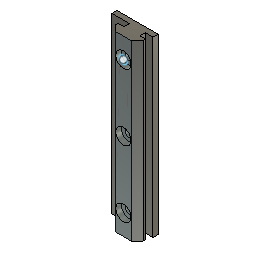
Slider v1 (Autodesk Fusion 360 design; units mm, degrees)
Autodesk Fusion 360 part; units mm, degrees
sketch "Sketch1" plane through (0, 0, 0) normal (0, 0, 1) x (1, 0, 0)
  line L0 (0, 0) -> (6.9, 0)
  line L1 (6.9, 0) -> (6.9, -2.1)
  line L2 (6.9, -2.1) -> (4.6, -2.1)
  line L3 (4.6, -2.1) -> (4.6, -3.1)
  line L4 (4.6, -3.1) -> (6.9335, -5.4335)
  line L5 (4.6, -3.1) -> (7.9, -3.1) construction
  line L6 (4.6, -2.1) -> (10.8, -2.1)
  line L7 (6.9, -2.1) -> (13.1, -2.1)
  line L8 (13.1, -2.1) -> (15.4, -2.1)
  line L9 (15.4, -2.1) -> (15.4, -3.1)
  line L10 (15.4, -3.1) -> (13.0665, -5.4335)
  line L11 (13.0665, -5.4335) -> (6.9335, -5.4335)
  line L12 (15.4, -2.1) -> (13.1, -2.1)
  line L13 (13.1, -2.1) -> (13.1, 0)
  line L14 (13.1, 0) -> (16.1, 0)
  line L15 (16.1, 0) -> (16.1, 2)
  line L16 (16.1, 2) -> (0, 2)
  line L17 (0, 2) -> (0, 0)
  dimension "d1" = 6.9
  dimension "d2" = 2.1
  dimension "d3" = 2.3
  dimension "d4" = 1
  dimension "d5" = 45
  dimension "d6" = 3.3
  dimension "d7" = 6.2
  dimension "d11" = 6.2
  dimension "d12" = 135
  dimension "d13" = 3.3
  dimension "d14" = 3
  constraint coincident L0.start L17.end
  constraint horizontal L0
  constraint perpendicular L0 L1
  constraint perpendicular L1 L2
  constraint perpendicular L2 L3
  constraint horizontal L5
  constraint perpendicular L3 L6
  constraint perpendicular L1 L7
  constraint parallel L7 L8
  constraint perpendicular L8 L9
  constraint perpendicular L12 L13
  constraint perpendicular L13 L14
  constraint perpendicular L14 L15
  constraint perpendicular L15 L16
  constraint perpendicular L0 L17
  measures "d1" distance of L0.start L0.end
  measures "d2" distance of L0.end L1.end
  measures "d3" distance of L1.end L2.end
  measures "d4" distance of L2.end L3.end
  measures "d5" angle of L4 L5
  measures "d6" distance of L3.end L4.end
  measures "d7" distance of L2.end L6.end
  measures "d11" distance of L1.end L7.end
  measures "d12" angle of L9 L10
  measures "d13" distance of L9.end L10.end
  measures "d14" distance of L13.end L14.end
extrude "Extrude1" add sketch "Sketch1" along normal blind 68
sketch "Sketch11" plane through (0, -5.4335, 0) normal (0, -1, 0) x (1, 0, 0)
  line L0 (6.9335, 0) -> (13.0665, 0)
  line L1 (13.0665, 0) -> (13.0665, 68)
  line L2 (13.0665, 68) -> (6.9335, 68)
  line L3 (6.9335, 68) -> (6.9335, 0)
  circle A0 centre (9.9608, 60) radius 1.475
  dimension "d119" = 2.95
  dimension "d126" = 8
  measures "d119" diameter of A0
  measures "d126" distance of L2 A0.centre
extrude "Extrude33" cut sketch "Sketch11" against normal blind 10 contours A0
pattern_linear "R-Pattern1" count 3 spacing 26 along (0, 0, -1) of "Extrude33"
sketch "Sketch12" plane through (0, -5.4335, 0) normal (0, -1, 0) x (1, 0, 0)
  circle A0 centre (9.9713, 60.0289) radius 3
  dimension "d127" = 6
  measures "d127" diameter of A0
extrude "Extrude34" cut sketch "Sketch12" against normal blind 2.2
pattern_linear "R-Pattern2" count 3 spacing 26 along (0, 0, -1) of "Extrude34"
